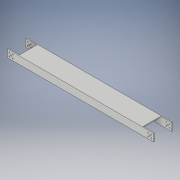
# Autodesk Inventor part: ArmProto2.2Assembly
Saved by Autodesk Inventor 2017 (Build 210142000, 142)
## iProperties
Created: 2017-10-04
Part Number: ArmProto2.2Assembly
Material: Generic
Document SubType Name: Modeling
Designer: User
Density: 1 g/cm^3
Appearance: Default
Author: User
Autodesk Inventor part; units mm, degrees
ref_plane "YZ Plane" through (0, 0, 0) normal (1, 0, 0) x (0, 1, 0)
ref_plane "XZ Plane" through (0, 0, 0) normal (0, 1, 0) x (-1, 0, 0)
ref_plane "XY Plane" through (0, 0, 0) normal (0, 0, 1) x (1, 0, 0)
sketch "Sketch1" plane through (0, 0, 0) normal (1, 0, 0) x (0, 1, 0)
  line L0 (0, 0) -> (25.4, 0)
  line L1 (25.4, 0) -> (25.4, -64.6049)
  line L2 (25.4, -64.6049) -> (0, -64.6049)
  line L3 (0, -64.6049) -> (0, 0)
  line L4 (0, -3.175) -> (22.225, -3.175)
  line L5 (22.225, -3.175) -> (22.225, -61.4299)
  line L6 (22.225, -61.4299) -> (0, -61.4299)
  line L7 (0, -61.4299) -> (0, -3.175)
  dimension "d0" = 25.4
  dimension "d2" = 58.2549
  dimension "d3" = 22.225
  dimension "d4" = 3.175
  dimension "d32" = 3.175
  constraints: 16 end point, 4 parallel, 2 horizontal, 2 perpendicular, 1 point on line
  measures "d0" distance of L1.end L2.end
  measures "d2" distance of L4.end L5.end
  measures "d3" distance of L5.end L6.end
  measures "d4" distance between parallel lines of L0 L4
  measures "d32" distance between parallel lines of L6 L2
extrude "Extrusion1" add sketch "Sketch1" along normal blind 495.3 contours L0 L1 L2 L3 L6 L5 L4
sketch "Sketch3" plane through (0, 25.4, 0) normal (0, 1, 0) x (1, 0, 0)
  line L0 (0, 64.6049) -> (0, 0) projected
  line L1 (0, 0) -> (495.3, 0) projected
  line L2 (495.3, 64.6049) -> (495.3, 0) projected
  line L3 (0, 64.6049) -> (495.3, 64.6049) projected
  line L4 (495.3, 3.175) -> (457.2, 3.175)
  line L5 (457.2, 3.175) -> (457.2, 61.4299)
  line L6 (457.2, 61.4299) -> (495.3, 61.4299)
  line L7 (495.3, 61.4299) -> (495.3, 3.175)
  line L8 (0, 64.6049) -> (0, 0) projected
  line L9 (0, 3.175) -> (38.1, 3.175)
  line L10 (38.1, 3.175) -> (38.1, 61.4299)
  line L11 (38.1, 61.4299) -> (0, 61.4299)
  line L12 (0, 61.4299) -> (0, 3.175)
  point P0 (495.3, 61.4299)
  dimension "d14" = 64.6049
  dimension "d16" = 38.1
  dimension "d27" = 38.1
  dimension "d28" = 58.2549
  dimension "d29" = 3.175
  dimension "d30" = 58.2549
  dimension "d31" = 3.175
  constraints: 16 end point, 4 parallel, 2 horizontal, 2 perpendicular, 2 point on line
  measures "d14" distance of L0.start L0.end
  measures "d16" distance of L5.end L6.end
  measures "d27" distance of L11.end L10.end
  measures "d28" distance of L9.end L10.end
  measures "d29" distance between parallel lines of L3 L11
  measures "d30" distance of L4.end L5.end
  measures "d31" distance between parallel lines of L3 L6
extrude "Extrusion2" cut sketch "Sketch3" against normal blind 3.175 contours L11 L10 L9 L0 | L2 L4 L5 L6
sketch "Sketch4" plane through (0, 0, 0) normal (0, 0, 1) x (1, 0, 0)
  line L0 (0, 25.4) -> (0, 0) projected
  line L1 (0, 0) -> (495.3, 0) projected
  line L2 (495.3, 25.4) -> (495.3, 0) projected
  line L3 (0, 25.4) -> (495.3, 25.4) projected
  circle A0 centre (12.7, 12.7) radius 2.3813
  circle A1 centre (482.6, 12.7) radius 2.3813
  line L4 (7.0485, 18.3515) -> (18.3515, 18.3515)
  line L5 (18.3515, 18.3515) -> (18.3515, 7.0485)
  line L6 (18.3515, 7.0485) -> (7.0485, 7.0485)
  line L7 (7.0485, 7.0485) -> (7.0485, 18.3515)
  line L8 (476.9485, 18.3515) -> (488.2515, 18.3515)
  line L9 (488.2515, 18.3515) -> (488.2515, 7.0485)
  line L10 (488.2515, 7.0485) -> (476.9485, 7.0485)
  line L11 (476.9485, 7.0485) -> (476.9485, 18.3515)
  dimension "d19" = 4.7625
  dimension "d20" = 12.7
  dimension "d21" = 25.4
  dimension "d22" = 12.7
  dimension "d23" = 4.7625
  dimension "d24" = 12.7
  dimension "d33" = 11.303
  dimension "d34" = 11.303
  dimension "d35" = 7.0485
  dimension "d36" = 7.0485
  dimension "d37" = 11.303
  dimension "d38" = 11.303
  dimension "d39" = 7.0485
  dimension "d40" = 7.0485
  constraints: 16 end point, 8 coincident, 4 parallel, 2 centre point, 2 horizontal, 2 perpendicular
  measures "d19" diameter of A0
  measures "d20" distance from line of L0 A0.centre
  measures "d21" distance of L0.start L0.end
  measures "d22" distance from line of L1 A0.centre
  measures "d23" diameter of A1
  measures "d24" distance from line of L2 A1.centre
  measures "d33" distance of L5.end L6.end
  measures "d34" distance of L4.end L5.end
  measures "d35" distance between parallel lines of L3 L4
  measures "d36" distance between parallel lines of L0 L7
  measures "d37" distance of L9.end L10.end
  measures "d38" distance of L8.end L9.end
  measures "d39" distance between parallel lines of L3 L8
  measures "d40" distance between parallel lines of L2 L9
extrude "Extrusion3" cut sketch "Sketch4" against normal blind 127 contours A0 | A1
sketch "Sketch5" plane through (0, 0, 0) normal (0, 0, 1) x (1, 0, 0)
  line L0 (0, 25.4) -> (0, 0)
  line L1 (0, 0) -> (495.3, 0)
  line L2 (495.3, 25.4) -> (495.3, 0)
  line L3 (0, 25.4) -> (495.3, 25.4)
  line L4 (7.0485, 18.3515) -> (18.3515, 18.3515)
  line L5 (18.3515, 18.3515) -> (18.3515, 7.0485)
  line L6 (18.3515, 7.0485) -> (7.0485, 7.0485)
  line L7 (7.0485, 7.0485) -> (7.0485, 18.3515)
  line L8 (476.9485, 18.3515) -> (488.2515, 18.3515)
  line L9 (488.2515, 18.3515) -> (488.2515, 7.0485)
  line L10 (488.2515, 7.0485) -> (476.9485, 7.0485)
  line L11 (476.9485, 7.0485) -> (476.9485, 18.3515)
  dimension "d43" = 25.4
  dimension "d47" = 11.303
  dimension "d48" = 11.303
  dimension "d49" = 7.0485
  dimension "d50" = 7.0485
  dimension "d51" = 11.303
  dimension "d52" = 11.303
  dimension "d53" = 7.0485
  dimension "d54" = 7.0485
  constraints: 24 end point, 8 coincident, 4 parallel, 2 horizontal, 2 perpendicular
  measures "d43" distance of L0.start L0.end
  measures "d47" distance of L5.end L6.end
  measures "d48" distance of L4.end L5.end
  measures "d49" distance between parallel lines of L3 L4
  measures "d50" distance between parallel lines of L0 L7
  measures "d51" distance of L9.end L10.end
  measures "d52" distance of L8.end L9.end
  measures "d53" distance between parallel lines of L3 L8
  measures "d54" distance between parallel lines of L2 L9
hole "Hole1" at (7.0485, 18.3515, 0) at (18.3515, 18.3515, 0) at (18.3515, 7.0485, 0) at (7.0485, 7.0485, 0) at (476.9485, 18.3515, 0) at (488.2515, 18.3515, 0) at (488.2515, 7.0485, 0) at (476.9485, 7.0485, 0) direction (0, 0, -1) diameter 3.5 depth 127 tip angle 118
equation "\"d32\" = d4"
equation "\"d30\" = d28"
equation "\"d31\" = d29"
equation "\"d22\" = 0.5 * d21"
equation "\"d23\" = d19"
equation "\"d24\" = d20"
equation "\"d35\" = -0.5 * d34 + 0.5 * d21"
equation "\"d36\" = d35"
equation "\"d37\" = d33"
equation "\"d38\" = d34"
equation "\"d39\" = d35"
equation "\"d40\" = d36"
equation "\"d49\" = -0.5 * d48 + 0.5 * d43"
equation "\"d50\" = d49"
equation "\"d51\" = d47"
equation "\"d52\" = d48"
equation "\"d53\" = d49"
equation "\"d54\" = d50"
body "Solid1"
